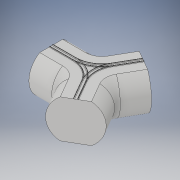
# Autodesk Inventor part: 3 way corridor
Saved by Autodesk Inventor 2017 (Build 210142000, 142)
## iProperties
Created: 2018-03-04
Part Number: 3 way corridor
Material: Generic
Document SubType Name: Modeling
Designer: Braxton
Density: 1 g/cm^3
Appearance: Default
Author: Braxton
Autodesk Inventor part; units mm, degrees
ref_plane "YZ Plane" through (0, 0, 0) normal (1, 0, 0) x (0, 1, 0)
ref_plane "XY Plane" through (0, 0, 0) normal (0, 0, 1) x (1, 0, 0)
sketch "Sketch1" plane through (0, 0, 0) normal (1, 0, 0) x (0, 1, 0)
  arc A0 (87.862241, -6.35) -> (84.666667, -3.154507) centre (84.687308, -6.32944) ccw construction
  arc A1 (84.666667, -4.084376) -> (86.913229, -6.35) centre (86.932372, -4.084376) ccw
  line L0 (87.862241, -7.408333) -> (86.254167, -7.408333)
  line L1 (87.862241, -7.408333) -> (87.862241, -6.35)
  arc A2 (86.254167, -7.408333) -> (84.666667, -8.995833) centre (86.254167, -8.995833) ccw
  arc A3 (84.666667, 50.8) -> (-84.666667, 50.8) centre (0, 0) ccw
  line L2 (84.666667, -8.995833) -> (84.666667, -50.8)
  arc A4 (-84.666667, -50.8) -> (84.666667, -50.8) centre (0, 0) ccw
  line L3 (-84.666667, 50.8) -> (-84.666667, -50.8)
  line L4 (84.687308, -6.32944) -> (87.862241, -3.154506) construction
  line L5 (87.862241, -6.35) -> (86.913229, -6.35)
  line L6 (87.862241, -6.35) -> (87.862241, 0) construction
  line L7 (87.862242, 7.408333) -> (86.254167, 7.408333)
  line L8 (84.666667, 8.995833) -> (84.666667, -8.995833) construction
  line L9 (84.666667, -4.084376) -> (84.666667, 0)
  line L10 (84.666667, 0) -> (87.862241, 0) construction
  line L11 (84.666667, 4.084376) -> (84.666667, 0)
  line L12 (87.862241, 6.35) -> (86.913229, 6.35)
  line L13 (87.862241, 6.35) -> (87.862241, 0) construction
  arc A5 (86.913229, 6.35) -> (84.666667, 4.084376) centre (86.932372, 4.084376) ccw
  line L14 (84.687308, 6.32944) -> (87.862241, 3.154506) construction
  arc A6 (84.666667, 3.154507) -> (87.862241, 6.35) centre (84.687308, 6.32944) ccw construction
  line L15 (87.862241, 6.35) -> (87.862242, 7.408333)
  line L16 (84.666667, 8.995833) -> (84.666667, 50.8)
  arc A7 (84.666667, 8.995833) -> (86.254167, 7.408333) centre (86.254167, 8.995833) ccw
  dimension "d105" = 101.6
  dimension "d106" = 14.81667
  dimension "d107" = 98.73745
  dimension "d108" = 98.73745
  dimension "d109" = 43.39167
  dimension "d110" = 1.5875
  dimension "d111" = 1.5875
  dimension "d112" = 41.80417
  dimension "d113" = 6.35
  dimension "d114" = 3.175
  dimension "d115" = 2.26571
  dimension "d116" = 2.24656
  dimension "d117" = 45
  dimension "d118" = 84.66667
  constraints: 34 end point, 19 point on circle, 8 centre point, 7 symmetric about line, 6 point on line, 5 collinear, 4 perpendicular, 3 coincident, 3 equal length, 2 tangent, 1 equal radius, 1 parallel, 1 vertical, 3 other
  measures "d105" distance of L16.end L2.end
  measures "d106" distance of L15.end L0.start
  measures "d107" radius of A3
  measures "d108" radius of A4
  measures "d109" distance from line of L16.end L7
  measures "d110" distance from line of L2.start L0
  measures "d111" radius of A2
  measures "d112" distance of L2.start L2.end
  measures "d113" distance of L6.end L13.start
  measures "d114" distance of L13.start L14.start
  measures "d115" radius of A5
  measures "d116" horizontal distance of L11.start L12.end
  measures "d117" angle of L13 L14
  measures "d118" distance from line of L3 point (0, 0)
extrude "corridor" add sketch "Sketch1" along normal blind 101.6
sketch "found rotaion axis" plane through (0, 0, 0) normal (0, 1, 0) x (-1, 0, 0)
  line L0 (-101.6, 124.137452) -> (-101.6, -124.137452)
  line L1 (-101.6, -124.137452) -> (-101.6, 124.137452)
  line L2 (-101.6, 0) -> (-173.270792, 0)
  point P0 (0, 0)
  dimension "d15" = 71.67079
  constraints: 4 end point, 1 horizontal, 1 midpoint, 1 vertical
  measures "d15" distance of L2.start L2.end
pattern_circular "other corridors" count 3 over 360 about axis through (173.270792, 0, 0) along (0, 1, 0) of "corridor"
sketch "Sketch5" plane through (101.6, 0, 0) normal (1, 0, 0) x (0, 0, -1)
  line L0 (-7.408333, 87.862242) -> (-7.408333, 86.254167)
  line L1 (-7.408333, 86.254167) -> (-7.408333, 87.862242)
  line L2 (-6.35, 86.913229) -> (-6.35, 87.862241)
  line L3 (-7.408333, 87.862242) -> (-6.35, 87.862241)
  line L4 (-6.35, 87.862241) -> (-6.35, 86.913229)
  arc A0 (-6.35, 86.913229) -> (-4.084376, 84.666667) centre (-4.084376, 86.932372) ccw
  arc A1 (4.084376, 84.666667) -> (6.35, 86.913229) centre (4.084376, 86.932372) ccw
  line L5 (4.084376, 84.666667) -> (-4.084376, 84.666667)
  line L6 (-4.084376, 84.666667) -> (4.084376, 84.666667)
  line L7 (6.35, 87.862241) -> (6.35, 86.913229)
  line L8 (6.35, 86.913229) -> (6.35, 87.862241)
  line L9 (7.408333, 87.862241) -> (6.35, 87.862241)
  line L10 (6.35, 87.862241) -> (7.408333, 87.862241)
  line L11 (7.408333, 86.254167) -> (7.408333, 87.862241)
  line L12 (7.408333, 87.862241) -> (7.408333, 86.254167)
  arc A2 (7.408333, 86.254167) -> (8.995833, 84.666667) centre (8.995833, 86.254167) ccw
  arc A3 (50.8, -84.666667) -> (50.8, 84.666667) centre (0, 0) ccw
  line L13 (50.8, 84.666667) -> (8.995833, 84.666667)
  line L14 (50.8, 84.666667) -> (8.995833, 84.666667)
  arc A4 (50.8, -84.666667) -> (50.8, 84.666667) centre (0, 0) ccw
  arc A5 (-8.995833, 84.666667) -> (-7.408333, 86.254167) centre (-8.995833, 86.254167) ccw
  arc A6 (-7.408333, 86.254167) -> (-7.408333, 86.254167) centre (-8.995833, 86.254167) ccw
  arc A7 (-6.35, 86.913229) -> (-4.084376, 84.666667) centre (-4.084376, 86.932372) ccw
  line L15 (-8.995833, 84.666667) -> (-50.8, 84.666667)
  arc A8 (-8.995833, 84.666667) -> (-7.408333, 86.254167) centre (-8.995834, 86.254167) ccw
  arc A9 (4.084376, 84.666667) -> (6.35, 86.913229) centre (4.084376, 86.932372) ccw
  arc A10 (7.408333, 86.254167) -> (8.995833, 84.666667) centre (8.995833, 86.254167) ccw
  arc A11 (-8.995833, 84.666667) -> (-7.408333, 86.254167) centre (-8.995833, 86.254167) ccw
  line L16 (-8.995833, 84.666667) -> (-8.995833, -84.666667)
  line L17 (-50.8, -84.666667) -> (50.8, -84.666667)
  line L18 (-8.995833, -84.666667) -> (50.8, -84.666667)
  constraints: 20 end point, 10 point on circle, 5 centre point, 5 concentric, 5 perpendicular, 3 collinear, 3 vertical, 2 tangent, 1 horizontal alignment, 1 point on line, 3 other
sketch "Sketch4" plane through (0, 0, 0) normal (0, 1, 0) x (-1, 0, 0)
  line L0 (0, -98.737452) -> (-101.6, -98.737452) construction
  line L1 (-174.397046, -199.425634) -> (-123.597046, -111.437453) construction
  line L2 (-345.41533, -100.688182) -> (-294.61533, -12.700001) construction
  line L3 (-345.41533, 100.688182) -> (-294.61533, 12.700001) construction
  line L4 (-174.397046, 199.425634) -> (-123.597046, 111.437453) construction
  line L5 (0, 98.737452) -> (-101.6, 98.737452) construction
  arc A0 (-101.6, -98.737452) -> (-123.597046, -111.437453) centre (-101.6, -124.137453) ccw
  arc A1 (-294.61533, -12.700001) -> (-294.61533, 12.700001) centre (-316.612376, 0) ccw
  line L6 (-165.112098, 87.468727) -> (-123.597046, 111.437453)
  line L7 (-101.6, 98.737452) -> (-101.6, 50.8)
  arc A2 (-123.597046, 111.437453) -> (-101.6, 98.737452) centre (-101.6, 124.137453) ccw
  constraints: 6 point on circle, 6 tangent, 3 centre point
sweep "curve edjes" add profiles "Sketch5" path "Sketch4" path curves A0 contours L3 L2 A0 L5 A1 L7 L9 L11 A2 L13 A3 L17 L16 A5 L0
pattern_circular "repeat curve edjes" count 3 over 360 about axis through (173.270792, 0, 0) along (0, 1, 0) of "curve edjes"
sketch "Sketch10" plane through (316.612376, 84.666667, 0) normal (0, 1, 0) x (1, 0, 0)
  arc A0 (-166.904532, 0) -> (-131.56011, 20.406111) centre (-215.012376, 124.137453) ccw
  arc A1 (-166.904532, 0) -> (-131.56011, 20.406111) centre (-215.012376, 124.137453) ccw
  arc A2 (-131.56011, 20.406111) -> (-131.56011, -20.406111) centre (0, 0) ccw
  arc A3 (-131.56011, 20.406111) -> (-131.56011, -20.406111) centre (0, 0) ccw
  arc A4 (-131.56011, -20.406111) -> (-166.904532, 0) centre (-215.012376, -124.137453) ccw
  arc A5 (-131.56011, -20.406111) -> (-166.904532, 0) centre (-215.012376, -124.137453) ccw
  point P0 (-316.612376, 0)
  constraints: 6 point on circle, 3 centre point, 3 concentric
extrude "hole fill in" add sketch "Sketch10" against normal up to surface (169.333333 mm away)
equation "\"d108\" = d107"
equation "\"d110\" = 0.5 * d119"
equation "\"d119\" = 3.175"
body "Solid1"
